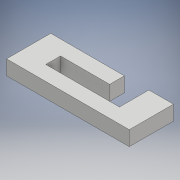
# Autodesk Inventor part: Zamkek_puszka
Saved by Autodesk Inventor 2018 (Build 220112000, 112)
## iProperties
Created: 2018-10-24
Part Number: Zamkek_puszka
Material: Ogólny
Document SubType Name: Modeling
Designer: EWA
Density: 1 g/cm^3
Appearance: Domyślna
Author: EWA
Autodesk Inventor part; units mm, degrees
ref_plane "YZ Plane" through (0, 0, 0) normal (1, 0, 0) x (0, 1, 0)
ref_plane "XZ Plane" through (0, 0, 0) normal (0, 1, 0) x (-1, 0, 0)
ref_plane "XY Plane" through (0, 0, 0) normal (0, 0, 1) x (1, 0, 0)
sketch "Szkic1" plane through (0, 0, 0) normal (0, 0, 1) x (1, 0, 0)
  line L0 (0, 0) -> (50, 0) construction
  line L1 (50, 0) -> (50, 18) construction
  line L2 (50, 18) -> (0, 18) construction
  line L3 (0, 18) -> (0, 0) construction
  line L4 (25, 18) -> (25, 0) construction
  line L5 (0, 0) -> (0, 6) construction
  line L6 (0, 6) -> (50, 6) construction
  line L7 (50, 6) -> (50, 12) construction
  line L8 (50, 12) -> (0, 12) construction
  line L9 (0, 12) -> (0, 6) construction
  line L10 (0, 18) -> (10, 18) construction
  line L11 (10, 18) -> (10, 0) construction
  line L12 (50, 18) -> (30, 18) construction
  line L13 (30, 18) -> (30, 0) construction
  line L14 (40, 18) -> (40, 0) construction
  line L15 (0, 0) -> (50, 0)
  line L16 (50, 0) -> (50, 18)
  line L17 (50, 18) -> (40, 18)
  line L18 (40, 18) -> (40, 6)
  line L19 (40, 6) -> (10, 6)
  line L20 (10, 6) -> (10, 12)
  line L21 (10, 12) -> (30, 12)
  line L22 (30, 12) -> (30, 18)
  line L23 (30, 18) -> (0, 18)
  line L24 (0, 18) -> (0, 0)
  dimension "d1" = 18
  dimension "d2" = 6
  dimension "d3" = 6
  dimension "d4" = 10
  dimension "d5" = 20
  dimension "d8" = 20
  constraints: 50 end point, 15 point on line, 7 perpendicular, 4 collinear, 4 parallel, 3 midpoint, 2 horizontal
  measures "d1" distance of L1.end L0.end
  measures "d2" distance of L0.start L5.end
  measures "d3" distance of L7.end L6.end
  measures "d4" distance of L2.end L10.end
  measures "d5" distance of L1.end L12.end
  measures "d8" distance of L12.end L10.end
extrude "Wyciągnięcie proste1" add sketch "Szkic1" along normal blind 6
